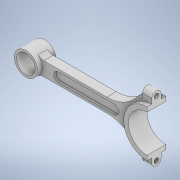
# Autodesk Inventor part: Ch4 Part 3
Saved by Autodesk Inventor 2020 (Build 240168000, 168)
## iProperties
Created: 2021-02-11
Part Number: Ch4 Part 3
Material: Generic
Document SubType Name: Modeling
Designer: austi
Density: 1 g/cm^3
Appearance: Default
Author: austi
Autodesk Inventor part; units mm, degrees
ref_plane "YZ Plane" through (0, 0, 0) normal (1, 0, 0) x (0, 1, 0)
ref_plane "XZ Plane" through (0, 0, 0) normal (0, 1, 0) x (-1, 0, 0)
ref_plane "XY Plane" through (0, 0, 0) normal (0, 0, 1) x (1, 0, 0)
sketch "Sketch1" plane through (0, 0, 0) normal (0, 0, 1) x (1, 0, 0)
  circle A0 centre (0, 0) radius 15.875
  dimension "d0" = 31.75
  constraints: 1 centre point, 1 coincident
  measures "d0" diameter of A0
extrude "Extrusion1" add sketch "Sketch1" along normal mid plane 25.4
sketch "Sketch2" plane through (0, 0, 0) normal (1, 0, 0) x (0, 1, 0)
  line L0 (0, 0) -> (9.525, 0)
  line L1 (9.525, 0) -> (9.525, -6.35)
  line L2 (9.525, -6.35) -> (-9.525, -6.35)
  line L3 (-9.525, -6.35) -> (-9.525, 6.35)
  line L4 (-9.525, 6.35) -> (9.525, 6.35)
  line L5 (9.525, 6.35) -> (9.525, 0)
  dimension "d3" = 9.525
  dimension "d4" = 6.35
  dimension "d5" = 19.05
  dimension "d6" = 12.7
  constraints: 12 end point, 5 perpendicular, 1 horizontal, 1 point on line
  measures "d3" distance of L0.start L0.end
  measures "d4" distance of L0.end L1.end
  measures "d5" distance of L1.end L2.end
  measures "d6" distance of L2.end L3.end
extrude "Extrusion2" add sketch "Sketch2" along normal blind 114.3
fillet "Fillet1" radius 12.7 3 edges at (12.7, 9.525, -3.175) (12.7, -9.525, -3.175) (12.7, -9.525, 3.175)
sketch "Sketch3" plane through (0, 0, 0) normal (0, 0, 1) x (1, 0, 0)
  point P0 (0, 0)
sketch "Sketch4" plane through (0, 0, 12.7) normal (0, 0, 1) x (1, 0, 0)
  point P0 (0, 0)
  point P1 (0, 0)
  constraints: 1 coincident
hole "Hole1" at (0, 0, 12.7) direction (0, 0, -1) diameter 25.4 depth 25.4 tip angle 118
sketch "Sketch7" plane through (0, 0, 0) normal (0, 0, 1) x (1, 0, 0)
  line L0 (114.3, 9.525) -> (114.3, -9.525) projected
  arc A0 (165.1, 25.4) -> (165.1, -25.4) centre (165.1, 0) ccw
  line L1 (165.1, 25.4) -> (165.1, 44.45)
  line L2 (165.1, 44.45) -> (152.4, 44.45)
  line L3 (152.4, 44.45) -> (152.4, 31.75)
  line L4 (152.4, 31.75) -> (146.05, 31.75)
  arc A1 (104.0487, 9.525) -> (146.05, 31.75) centre (104.0487, 60.325) ccw
  line L5 (17.9605, 9.525) -> (114.3, 9.525) projected
  line L6 (165.1, -25.4) -> (165.1, -44.45)
  line L7 (165.1, -44.45) -> (152.4, -44.45)
  line L8 (152.4, -44.45) -> (152.4, -31.75)
  line L9 (152.4, -31.75) -> (146.05, -31.75)
  arc A2 (146.05, -31.75) -> (104.0487, -9.525) centre (104.0487, -60.325) ccw
  line L10 (0, -84.455) -> (0, 84.455) projected
  line L11 (-52.07, 0) -> (201.295, 0) projected
  line L12 (17.9605, -9.525) -> (114.3, -9.525) projected
  point P0 (0, 0)
  point P1 (139.7, 0)
  dimension "d40" = 19.05
  dimension "d41" = 12.7
  dimension "d42" = 12.7
  dimension "d43" = 6.35
  dimension "d45" = 25.4
  dimension "d46" = 50.8
  dimension "d47" = 19.05
  dimension "d48" = 88.9
  dimension "d49" = 165.1
  constraints: 16 end point, 7 point on circle, 4 perpendicular, 3 centre point, 1 line through centre, 1 parallel, 1 point on line, 1 tangent, 5 other
  measures "d40" distance of L1.start L1.end
  measures "d41" distance of L1.end L2.end
  measures "d42" distance of L2.end L3.end
  measures "d43" distance of L3.end L4.end
  measures "d45" radius of A0
  measures "d46" radius of A1
  measures "d47" distance from line of L12 A1.start
  measures "d48" distance of L7.start L1.end
  measures "d49" horizontal distance of point (0, 0) L7.start
extrude "Extrusion3" add sketch "Sketch7" along normal mid plane 12.7
sketch "Sketch11" plane through (0, 0, 6.35) normal (0, 0, 1) x (1, 0, 0)
  arc A0 (165.1, 31.75) -> (165.1, -31.75) centre (165.1, 0) ccw
  arc A1 (165.1, 25.4) -> (165.1, -25.4) centre (165.1, 0) ccw projected
  arc A2 (165.1, 25.4) -> (165.1, -25.4) centre (165.1, 0) ccw
  line L0 (165.1, 25.4) -> (165.1, 44.45) projected
  line L1 (165.1, 31.75) -> (165.1, 25.4)
  line L2 (165.1, -44.45) -> (165.1, -25.4) projected
  line L3 (165.1, -25.4) -> (165.1, -31.75)
  point P0 (0, 0)
  dimension "d56" = 25.4
  dimension "d57" = 31.75
  constraints: 4 end point, 4 point on circle, 2 centre point, 2 point on line, 1 coincident, 1 collinear, 1 concentric
  measures "d56" radius of A1
  measures "d57" radius of A0
extrude "Extrusion5" add sketch "Sketch11" along normal blind 6.35
sketch "Sketch12" plane through (0, 0, -6.35) normal (0, 0, -1) x (-1, 0, 0)
  arc A0 (-165.1, -25.4) -> (-165.1, 25.4) centre (-165.1, 0) ccw projected
  arc A1 (-165.1, -25.4) -> (-165.1, 25.4) centre (-165.1, 0) ccw
  arc A2 (-165.1, -31.75) -> (-165.1, 31.75) centre (-165.1, 0) ccw
  line L0 (-165.1, 44.45) -> (-165.1, 25.4) projected
  line L1 (-165.1, 31.75) -> (-165.1, 25.4)
  line L2 (-165.1, -31.75) -> (-165.1, -25.4) projected
  line L3 (-165.1, -25.4) -> (-165.1, -31.75)
  point P0 (0, 0)
  constraints: 4 end point, 4 point on circle, 2 centre point, 2 coincident, 2 collinear
extrude "Extrusion6" add sketch "Sketch12" along normal blind 6.35
sketch "Sketch13" plane through (165.1, 44.45, 6.35) normal (1, 0, 0) x (0, 0, -1)
  point P0 (6.35, -44.45)
  point P1 (6.35, -6.35)
  point P2 (6.35, -82.55)
hole "Hole2" at (165.1, 38.1, 0) at (165.1, -38.1, 0) direction (-1, 0, 0) diameter 6.35 depth 12.7 tip angle 118
fillet "Fillet2" radius 6.35 4 edges at (158.75, 44.45, 6.35) (158.75, 44.45, -6.35) (158.75, -44.45, 6.35) (158.75, -44.45, -6.35)
sketch "Sketch14" plane through (0, 0, 6.35) normal (0, 0, 1) x (1, 0, 0)
  line L0 (17.9605, -9.525) -> (104.0487, -9.525) projected
  line L1 (0, -62.23) -> (0, 62.23) projected
  arc A0 (38.1, 6.35) -> (38.1, -6.35) centre (38.1, 0) ccw
  line L2 (38.1, 6.35) -> (114.3, 6.35)
  line L3 (38.1, -6.35) -> (114.3, -6.35)
  arc A1 (114.3, -6.35) -> (114.3, 6.35) centre (114.3, 0) ccw
  point P0 (0, 0)
  dimension "d73" = 12.7
  dimension "d74" = 76.2
  dimension "d75" = 76.2
  dimension "d76" = 12.7
  dimension "d77" = 38.1
  constraints: 4 end point, 4 point on circle, 2 centre point, 2 horizontal, 1 equal radius, 1 horizontal alignment, 1 tangent
  measures "d73" diameter of A0
  measures "d74" distance of L2.start L2.end
  measures "d75" distance of L3.end L3.start
  measures "d76" distance between parallel lines of L3 L2
  measures "d77" distance of A0.centre point (0, 0)
extrude "Extrusion7" cut sketch "Sketch14" against normal blind 3.175
sketch "Sketch15" plane through (0, 0, -6.35) normal (0, 0, -1) x (-1, 0, 0)
  line L0 (0, 0) -> (-38.1, 0)
  arc A0 (-38.1, -6.35) -> (-38.1, 6.35) centre (-38.1, 0) ccw
  line L1 (-38.1, 6.35) -> (-114.3, 6.35)
  line L2 (-38.1, 6.35) -> (-114.3, 6.35)
  line L3 (-114.3, -6.35) -> (-38.1, -6.35) projected
  line L4 (-38.1, -6.35) -> (-114.3, -6.35)
  arc A1 (-114.3, 6.35) -> (-114.3, -6.35) centre (-114.3, 0) ccw
  dimension "d80" = 38.1
  dimension "d82" = 76.2
  constraints: 9 end point, 4 point on circle, 2 centre point, 2 equal length, 2 horizontal, 1 coincident, 1 equal radius, 1 other
  measures "d80" distance of L0.start L0.end
  measures "d82" distance of L1.start L1.end
extrude "Extrusion8" cut sketch "Sketch15" against normal blind 3.175
body "Solid1"
